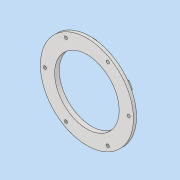
# Autodesk Inventor part: forwardBallastSealingWallRear
Saved by Autodesk Inventor 2017 (Build 210142000, 142)
## iProperties
Created: 2016-11-26
Part Number: forwardBallastSealingWallRear
Material: ABS Plastic
Document SubType Name: Modeling
Designer: techn
Density: 1.06 g/cm^3
Appearance: Smooth - White
Author: techn
Autodesk Inventor part; units mm, degrees
ref_plane "YZ Plane" through (0, 0, 0) normal (1, 0, 0) x (0, 1, 0)
ref_plane "XZ Plane" through (0, 0, 0) normal (0, 1, 0) x (-1, 0, 0)
ref_plane "XY Plane" through (0, 0, 0) normal (0, 0, 1) x (1, 0, 0)
sketch "Sketch1" plane through (0, 0, 0) normal (0, 0, 1) x (1, 0, 0)
  circle A0 centre (0, 0) radius 47.625
  line L0 (0, 0) -> (21.4313, 37.12)
  line L1 (0, 0) -> (42.8625, 0) construction
  circle A1 centre (21.4313, 37.12) radius 1.5875
  circle A2 centre (-21.4312, 37.12) radius 1.5875
  circle A3 centre (-42.8625, 0) radius 1.5875
  circle A4 centre (-21.4313, -37.12) radius 1.5875
  circle A5 centre (21.4312, -37.12) radius 1.5875
  circle A6 centre (42.8625, 0) radius 1.5875
  dimension "d0" = 95.25
  dimension "d1" = 42.8625
  dimension "d2" = 60
  dimension "d3" = 3.175
  dimension "d6" = 360
  constraints: 7 centre point, 4 end point, 2 coincident, 1 equal length, 1 horizontal, 13 other
  measures "d0" diameter of A0
  measures "d1" distance of L0.start L0.end
  measures "d2" angle of L1 L0
  measures "d3" diameter of A1
extrude "Extrusion1" add sketch "Sketch1" along normal blind 3.175
sketch "Sketch3" plane through (0, 0, 0) normal (0, 0, -1) x (-1, 0, 0)
  circle A0 centre (0, 0) radius 41.275
  circle A1 centre (0, 0) radius 34.925
  dimension "d10" = 82.55
  dimension "d11" = 69.85
  constraints: 2 centre point, 2 coincident
  measures "d10" diameter of A0
  measures "d11" diameter of A1
extrude "Extrusion2" add sketch "Sketch3" along normal blind 1.5875 contours A1
sketch "Sketch5" plane through (0, 0, 0) normal (0, 0, -1) x (-1, 0, 0)
  circle A0 centre (0, 0) radius 41.275
  line L0 (0, 0) -> (37.4079, 17.4436)
  line L1 (0, 0) -> (41.275, 0) construction
  line L2 (0, 0) -> (33.8105, 23.6744)
  line L3 (0, 0) -> (41.275, 0) construction
  line L4 (37.4079, 17.4436) -> (40.2854, 18.7854)
  line L5 (33.8105, 23.6744) -> (36.4113, 25.4955)
  arc A1 (40.2854, 18.7854) -> (36.4113, 25.4955) centre (0, 0) ccw
  arc A2 (37.4079, 17.4436) -> (33.8105, 23.6744) centre (0, 0) ccw
  dimension "d14" = 82.55
  dimension "d15" = 41.275
  dimension "d16" = 25
  dimension "d17" = 41.275
  dimension "d18" = 35
  dimension "d19" = 3.175
  dimension "d20" = 3.175
  dimension "d21" = 44.45
  constraints: 12 end point, 4 point on circle, 3 centre point, 2 equal length, 2 horizontal, 1 coincident, 1 concentric
  measures "d14" diameter of A0
  measures "d15" distance of L0.start L0.end
  measures "d16" angle of L1 L0
  measures "d17" distance of L0.start L2.end
  measures "d18" angle of L3 L2
  measures "d19" distance of L0.end L4.end
  measures "d20" distance of L2.end L5.end
  measures "d21" radius of A1
extrude "Extrusion3" add sketch "Sketch5" along normal blind 3.175 contours A0 L5 A1 L4
pattern_circular "Circular Pattern1" count 6 over 360 about axis through (0, 0, 0) along (0, 0, 1) of "Extrusion3"
sketch "Sketch6" plane through (0, 0, -1.5875) normal (0, 0, -1) x (-1, 0, 0)
  circle A0 centre (0, 0) radius 33.02
  dimension "d27" = 66.04
  constraints: 1 centre point, 1 coincident
  measures "d27" diameter of A0
extrude "Extrusion4" cut sketch "Sketch6" against normal blind 25.4
body "Solid1"
